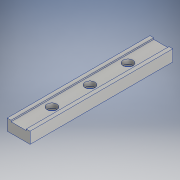
# Autodesk Inventor part: LR Small Clamp
Saved by Autodesk Inventor 2019 (Build 230136000, 136)
## iProperties
Created: 2016-01-25
Part Number: LR Small Clamp
Material: Aluminum 6061
Document SubType Name: Modeling
Designer: IEUser
Density: 2.7 g/cm^3
Appearance: Aluminum - Flat
Mass: 11.771 g
Surface Area: 30.197 cm^2
Volume: 4.35963 cm^3
Author: IEUser
Autodesk Inventor part; units mm, degrees
ref_plane "YZ Plane" through (0, 0, 0) normal (1, 0, 0) x (0, 1, 0)
ref_plane "XZ Plane" through (0, 0, 0) normal (0, 1, 0) x (-1, 0, 0)
ref_plane "XY Plane" through (0, 0, 0) normal (0, 0, 1) x (1, 0, 0)
sketch "Body Outline" plane through (0, 0, 0) normal (0, 1, 0) x (-1, 0, 0)
  line L0 (37.5, -6) -> (-37.5, -6)
  line L1 (-37.5, -6) -> (-37.5, 6)
  line L2 (-37.5, 6) -> (37.5, 6)
  line L3 (37.5, 6) -> (37.5, -6)
  point P0 (0, 0)
  dimension "d0" = 75
  dimension "d1" = 37.5
  dimension "d2" = 12
  dimension "d3" = 6
  constraints: 8 end point, 2 parallel, 1 horizontal, 1 perpendicular
  measures "d0" distance of L0.start L0.end
  measures "d1" distance from line of point (0, 0) L3
  measures "d2" distance of L2.end L0.start
  measures "d3" distance from line of point (0, 0) L0
extrude "Body" add sketch "Body Outline" along normal blind 6
sketch "Clamp Cutout Outline" plane through (37.5, 0, 6) normal (1, 0, 0) x (0, 0, -1)
  line L0 (2, 7.3) -> (10, 7.3)
  line L1 (10, 7.3) -> (10, 5.3)
  line L2 (10, 5.3) -> (2, 5.3)
  line L3 (2, 5.3) -> (2, 7.3)
  line L4 (0, 6) -> (12, 6) projected
  line L5 (0, 0) -> (0, 6) projected
  line L6 (12, 0) -> (12, 6) projected
  point P0 (6, 0)
  dimension "d6" = 0.7
  dimension "d7" = 2
  dimension "d8" = 2
  dimension "d9" = 2
  constraints: 8 end point, 2 parallel, 1 horizontal, 1 perpendicular
  measures "d6" distance between parallel lines of L4 L2
  measures "d7" distance between parallel lines of L5 L3
  measures "d8" distance between parallel lines of L6 L1
  measures "d9" distance of L2.end L0.start
extrude "Clamp Cutout" cut sketch "Clamp Cutout Outline" along normal through all both and the other way through all
sketch "Fastening Hole Positions" plane through (0, 0, 0) normal (0, -1, 0) x (1, 0, 0)
  point P0 (0, 0)
  point P1 (20, 0)
  point P2 (0, 0)
  point P3 (-20, 0)
  dimension "d12" = 20
  dimension "d13" = 20
  dimension "d14" = 0
  dimension "d15" = 0
  dimension "d16" = 0
  dimension "d17" = 0
  measures "d12" distance of point (20, 0) point (0, 0)
  measures "d13" distance of point (-20, 0) point (0, 0)
  measures "d14" distance of point (0, 0) point (0, 0)
  measures "d15" vertical distance of point (0, 0) point (20, 0)
  measures "d16" distance of point (0, 0) point (0, 0)
  measures "d17" vertical distance of point (0, 0) point (-20, 0)
hole "Fastening Holes" at (20, 0, 0) at (0, 0, 0) at (-20, 0, 0) direction (0, 1, 0) diameter 5.2 end through all countersink diameter 11 countersink angle 90
equation "\"d1\" = 0.5 * d0"
equation "\"d3\" = 0.5 * d2"
equation "\"d8\" = d7"
body "Solid1"
